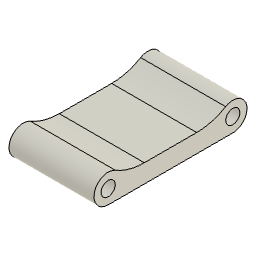
wing frame with feathers [both L + R] (Autodesk Fusion 360 archive; units mm, degrees)
design "pivots"
Autodesk Fusion 360 part; units mm, degrees
sketch "Sketch1" plane through (0, 0, 0) normal (1, 0, 0) x (0, 1, 0)
  line L0 (0, 0) -> (17, 0)
  circle A0 centre (20, 2.5) radius 1.25
  line L1 (-2, 0) -> (20, 0)
  line L2 (13.6213, 3.25) -> (4.3787, 3.25)
  arc A1 (-0.7243, 4.65) -> (-2, 0) centre (-2, 2.5) ccw
  arc A2 (20, 0) -> (18.7243, 4.65) centre (20, 2.5) ccw
  arc A3 (-0.7243, 4.65) -> (4.3787, 3.25) centre (4.3787, 13.25) ccw
  arc A4 (13.6213, 3.25) -> (18.7243, 4.65) centre (13.6213, 13.25) ccw
  circle A5 centre (-2, 2.5) radius 1.25
  dimension "d1" = 17
  dimension "d7" = 2.5
  dimension "d8" = 10
  dimension "d11" = 2.5
  constraint horizontal L0
  constraint coincident L0.start origin
  constraint concentric A0 A2
  constraint tangent L1 A2
  constraint parallel L0 L1
  constraint tangent L2 A3
  constraint tangent A1 A3
  constraint tangent L2 A4
  constraint tangent A2 A4
  constraint equal A3 A4
  constraint concentric A1 A5
  measures "d1" distance of L0.start L0.end
  measures "d7" diameter of A0
  measures "d8" radius of A3
  measures "d11" diameter of A5
extrude "Extrude1" add sketch "Sketch1" along normal blind 20 contours L0 L1 L2 A1 A2 A3 A4 | A0 | A5
extrude "Extrude2" cut sketch "Sketch1" along normal blind 50 contours A0
extrude "Extrude3" cut sketch "Sketch1" along normal blind 25.474 contours A5
extrude "Extrude4" cut 1 faces at (20, 7.4596, 1.0833) along direction (-1, 0, 0) blind 5
equation "d1 = 2 mm + 13 mm + 2 mm"

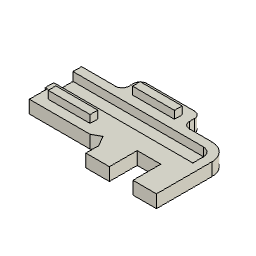
design "Right Shoulder Top"
Autodesk Fusion 360 part; units mm, degrees
sketch "Sketch1" plane through (0, 0, 0) normal (0, 0, 1) x (1, 0, 0)
  line L0 (0, 0) -> (20, 0)
  line L1 (20, 0) -> (20, 4.5)
  line L2 (20, 4.5) -> (0, 4.5)
  line L3 (0, 4.5) -> (0, 0)
  line L4 (20, 0) -> (21.5, 0)
  line L5 (21.5, 0) -> (21.5, 15)
  line L6 (21.5, 15) -> (20, 15)
  line L7 (20, 15) -> (20, 0)
  line L8 (31, 0) -> (32.5, 0)
  line L9 (32.5, 0) -> (32.5, 15)
  line L10 (32.5, 15) -> (31, 15)
  line L11 (31, 15) -> (31, 0)
  line L12 (20, 4.5) -> (16, 4.5)
  line L13 (16, 4.5) -> (16, 11.5)
  line L14 (16, 11.5) -> (20, 11.5)
  line L15 (20, 11.5) -> (20, 4.5)
  line L16 (21.5, 0) -> (31, 0)
  line L17 (31, 0) -> (31, 4.5)
  line L18 (31, 4.5) -> (21.5, 4.5)
  line L19 (21.5, 4.5) -> (21.5, 0)
  line L20 (21.5, 4.5) -> (31, 4.5)
  line L21 (31, 4.5) -> (31, 9.5)
  line L22 (31, 9.5) -> (21.5, 9.5)
  line L23 (21.5, 9.5) -> (21.5, 4.5)
  line L24 (81, 15) -> (81, 9.5)
  line L25 (50, 0) -> (70, 0)
  line L26 (71.5, 15) -> (70, 15)
  line L27 (50, 4.5) -> (50, 0)
  line L28 (66, 4.5) -> (50, 4.5)
  line L29 (82.5, 2) -> (82.5, 15)
  line L30 (71.5, 0) -> (80.5, 0)
  line L31 (82.5, 15) -> (81, 15)
  line L32 (70, 15) -> (70, 11.5)
  line L33 (70, 0) -> (71.5, 0)
  line L34 (71.5, 9.5) -> (71.5, 15)
  line L35 (66, 4.5) -> (70, 11.5)
  line L36 (71.5, 9.5) -> (71.5, 6.5)
  line L37 (71.5, 6.5) -> (81, 6.5)
  line L38 (81, 6.5) -> (81, 9.5)
  arc A0 (80.5, 0) -> (82.5, 2) centre (80.5, 2) ccw
  line L39 (70, -2) -> (71.5, -2)
  arc A1 (80.5, -2) -> (84.5, 2) centre (80.5, 2) ccw
  line L40 (84.5, 2) -> (84.5, 15)
  line L41 (79, 15) -> (79, 9.5)
  line L42 (79, 8.5) -> (79, 9.5)
  line L43 (73.5, 8.5) -> (79, 8.5)
  line L44 (73.5, 9.5) -> (73.5, 8.5)
  line L45 (73.5, 9.5) -> (73.5, 15)
  line L46 (68, 15) -> (68, 12.0311)
  line L47 (66.6143, 9.6061) -> (68, 12.0311)
  line L48 (50, 6.5) -> (50, -2)
  line L49 (68, 15) -> (73.5, 15)
  line L50 (79, 15) -> (84.5, 15)
  line L51 (52.5, 6.5) -> (62.7, 6.5)
  line L52 (62.7, 6.5) -> (62.7, 8.7)
  line L53 (62.7, 8.7) -> (52.5, 8.7)
  line L54 (52.5, 8.7) -> (52.5, 6.5)
  line L55 (64.7, 10.7) -> (50.5, 10.7)
  line L56 (50.5, 10.7) -> (50.5, 6.5)
  line L57 (62.7, 6.5) -> (52.5, 6.5)
  line L58 (50.5, 6.5) -> (50, 6.5)
  line L59 (64.7, 10.7) -> (66.6143, 9.6061)
  line L60 (61.5, -2) -> (71.7, -2)
  line L61 (71.7, -2) -> (71.7, -4.2)
  line L62 (71.7, -4.2) -> (61.5, -4.2)
  line L63 (61.5, -4.2) -> (61.5, -2)
  line L64 (73.7, -3.5) -> (73.7, -4.7)
  line L65 (72.2, -6.2) -> (61, -6.2)
  line L66 (59.5, -4.7) -> (59.5, -3.5)
  line L67 (71.5, -2) -> (71.7, -2)
  line L68 (75.2, -2) -> (80.5, -2)
  line L69 (50, -2) -> (58, -2)
  line L70 (61.5, -2) -> (70, -2)
  arc A2 (75.2, -2) -> (73.7, -3.5) centre (75.2, -3.5) ccw
  arc A3 (72.2, -6.2) -> (73.7, -4.7) centre (72.2, -4.7) ccw
  arc A4 (59.5, -4.7) -> (61, -6.2) centre (61, -4.7) ccw
  arc A5 (59.5, -3.5) -> (58, -2) centre (58, -3.5) ccw
  line L71 (70, 15) -> (71.5, 15)
  line L72 (71.5, 15) -> (71.5, 11.5)
  line L73 (71.5, 11.5) -> (70, 11.5)
  line L74 (70, 11.5) -> (70, 15)
  line L75 (71.7, -2) -> (71.7, -4.2)
  line L76 (61.5, -2) -> (71.7, -2)
  line L77 (70, -2) -> (71.5, -2)
  line L78 (71.7, -4.2) -> (61.5, -4.2)
  line L79 (68, 15) -> (73.5, 15)
  line L80 (70, 15) -> (71.5, 15)
  line L81 (71.5, 11.5) -> (70, 11.5)
  line L82 (72.2, -6.2) -> (61, -6.2)
  line L83 (71.5, 15) -> (70, 15)
  line L84 (70, 0) -> (71.5, 0)
  line L85 (71.5, 9.5) -> (71.5, 15)
  line L86 (73.5, 8.5) -> (79, 8.5)
  line L87 (70, 15) -> (70, 11.5)
  line L88 (75.2, -2) -> (80.5, -2)
  line L89 (79, 8.5) -> (79, 9.5)
  line L90 (82.5, 15) -> (81, 15)
  line L91 (81, 15) -> (81, 9.5)
  line L92 (73.5, 9.5) -> (73.5, 8.5)
  line L93 (71.5, 6.5) -> (81, 6.5)
  arc A6 (75.2, -2) -> (73.7, -3.5) centre (75.2, -3.5) ccw
  arc A7 (80.5, -2) -> (84.5, 2) centre (80.5, 2) ccw
  line L94 (61.5, -2) -> (70, -2)
  line L95 (71.5, 15) -> (71.5, 11.5)
  line L96 (52.5, 8.7) -> (52.5, 6.5)
  line L97 (52.5, 6.5) -> (62.7, 6.5)
  line L98 (79, 15) -> (79, 9.5)
  line L99 (68, 15) -> (68, 12.0311)
  line L100 (82.5, 2) -> (82.5, 15)
  line L101 (66, 4.5) -> (50, 4.5)
  line L102 (79, 15) -> (84.5, 15)
  line L103 (50, 4.5) -> (50, 0)
  line L104 (64.7, 10.7) -> (66.6143, 9.6061)
  line L105 (73.5, 9.5) -> (73.5, 15)
  line L106 (50.5, 10.7) -> (50.5, 6.5)
  line L107 (50, 0) -> (70, 0)
  line L108 (84.5, 2) -> (84.5, 15)
  line L109 (59.5, -4.7) -> (59.5, -3.5)
  line L110 (71.5, -2) -> (71.7, -2)
  line L111 (61.5, -4.2) -> (61.5, -2)
  line L112 (73.7, -3.5) -> (73.7, -4.7)
  line L113 (50, 6.5) -> (50, -2)
  line L114 (71.5, 0) -> (80.5, 0)
  arc A8 (59.5, -4.7) -> (61, -6.2) centre (61, -4.7) ccw
  line L115 (81, 6.5) -> (81, 9.5)
  arc A9 (59.5, -3.5) -> (58, -2) centre (58, -3.5) ccw
  line L116 (62.7, 8.7) -> (52.5, 8.7)
  arc A10 (72.2, -6.2) -> (73.7, -4.7) centre (72.2, -4.7) ccw
  line L117 (70, 11.5) -> (70, 15)
  arc A11 (80.5, 0) -> (82.5, 2) centre (80.5, 2) ccw
  line L118 (50.5, 6.5) -> (50, 6.5)
  line L119 (66.6143, 9.6061) -> (68, 12.0311)
  line L120 (71.5, 9.5) -> (71.5, 6.5)
  line L121 (62.7, 6.5) -> (52.5, 6.5)
  line L122 (64.7, 10.7) -> (50.5, 10.7)
  line L123 (50, -2) -> (58, -2)
  line L124 (62.7, 6.5) -> (62.7, 8.7)
  line L125 (66, 4.5) -> (70, 11.5)
  line L126 (50, 42) -> (58, 42)
  line L127 (66.6143, 30.3939) -> (68, 27.9689)
  line L128 (50.5, 33.5) -> (50, 33.5)
  line L129 (50, 33.5) -> (50, 42)
  line L130 (64.7, 29.3) -> (66.6143, 30.3939)
  line L131 (64.7, 29.3) -> (50.5, 29.3)
  line L132 (68, 25) -> (68, 27.9689)
  line L133 (50, 40) -> (70, 40)
  line L134 (50, 35.5) -> (50, 40)
  line L135 (50.5, 33.5) -> (50, 33.5)
  line L136 (50, 42) -> (58, 42)
  arc A12 (61, 46.2) -> (59.5, 44.7) centre (61, 44.7) ccw
  line L137 (64.7, 29.3) -> (50.5, 29.3)
  arc A13 (58, 42) -> (59.5, 43.5) centre (58, 43.5) ccw
  line L138 (50.5, 29.3) -> (50.5, 33.5)
  line L139 (59.5, 44.7) -> (59.5, 43.5)
  line L140 (73.5, 30.5) -> (73.5, 25)
  line L141 (70, 40) -> (71.5, 40)
  line L142 (79, 31.5) -> (79, 30.5)
  line L143 (50, 33.5) -> (50, 42)
  line L144 (71.5, 40) -> (80.5, 40)
  line L145 (66.6143, 30.3939) -> (68, 27.9689)
  line L146 (66, 35.5) -> (50, 35.5)
  line L147 (64.7, 29.3) -> (66.6143, 30.3939)
  arc A14 (82.5, 38) -> (80.5, 40) centre (80.5, 38) ccw
  line L148 (50, 35.5) -> (50, 40)
  line L149 (50, 40) -> (70, 40)
  line L150 (84.5, 38) -> (84.5, 25)
  line L151 (79, 25) -> (84.5, 25)
  line L152 (79, 25) -> (79, 30.5)
  line L153 (68, 25) -> (73.5, 25)
  line L154 (73.5, 31.5) -> (79, 31.5)
  line L155 (79, 25) -> (79, 30.5)
  line L156 (70, 25) -> (71.5, 25)
  line L157 (68, 25) -> (73.5, 25)
  line L158 (71.5, 25) -> (70, 25)
  line L159 (75.2, 42) -> (80.5, 42)
  line L160 (70, 25) -> (71.5, 25)
  arc A15 (73.7, 44.7) -> (72.2, 46.2) centre (72.2, 44.7) ccw
  arc A16 (84.5, 38) -> (80.5, 42) centre (80.5, 38) ccw
  line L161 (73.7, 43.5) -> (73.7, 44.7)
  line L162 (73.5, 30.5) -> (73.5, 31.5)
  line L163 (73.5, 30.5) -> (73.5, 31.5)
  line L164 (79, 25) -> (84.5, 25)
  line L165 (82.5, 25) -> (81, 25)
  arc A17 (73.7, 43.5) -> (75.2, 42) centre (75.2, 43.5) ccw
  line L166 (73.7, 43.5) -> (73.7, 44.7)
  line L167 (71.5, 40) -> (80.5, 40)
  line L168 (79, 31.5) -> (79, 30.5)
  line L169 (71.5, 25) -> (70, 25)
  line L170 (82.5, 25) -> (81, 25)
  line L171 (75.2, 42) -> (80.5, 42)
  line L172 (70, 40) -> (71.5, 40)
  line L173 (72.2, 46.2) -> (61, 46.2)
  line L174 (73.5, 31.5) -> (79, 31.5)
  line L175 (73.5, 30.5) -> (73.5, 25)
  line L176 (72.2, 46.2) -> (61, 46.2)
  arc A18 (73.7, 43.5) -> (75.2, 42) centre (75.2, 43.5) ccw
  arc A19 (58, 42) -> (59.5, 43.5) centre (58, 43.5) ccw
  arc A20 (82.5, 38) -> (80.5, 40) centre (80.5, 38) ccw
  arc A21 (84.5, 38) -> (80.5, 42) centre (80.5, 38) ccw
  line L177 (68, 25) -> (68, 27.9689)
  arc A22 (73.7, 44.7) -> (72.2, 46.2) centre (72.2, 44.7) ccw
  line L178 (59.5, 44.7) -> (59.5, 43.5)
  line L179 (50.5, 29.3) -> (50.5, 33.5)
  arc A23 (61, 46.2) -> (59.5, 44.7) centre (61, 44.7) ccw
  line L180 (66, 35.5) -> (50, 35.5)
  line L181 (84.5, 38) -> (84.5, 25)
  line L182 (52.7, 31.5) -> (52.7, 33.3)
  line L183 (62.5, 33.3) -> (52.7, 33.3)
  line L184 (62.5, 33.3) -> (62.5, 31.5)
  line L185 (62.5, 31.5) -> (52.7, 31.5)
  line L186 (71.5, 42.2) -> (71.5, 44)
  line L187 (71.5, 44) -> (61.7, 44)
  line L188 (61.7, 44) -> (61.7, 42.2)
  line L189 (61.7, 42.2) -> (71.5, 42.2)
  line L190 (66, 35.5) -> (82.5, 35.5)
  line L191 (82.5, 38) -> (82.5, 35.5)
  point P0 (50, 0)
  point P1 (50, 0)
  point P2 (50, 40)
  point P3 (50, 40)
  dimension "d1" = 20
  dimension "d2" = 4.5
  dimension "d3" = 1.5
  dimension "d4" = 15
  dimension "d5" = 1.5
  dimension "d6" = 15
  dimension "d7" = 9.5
  dimension "d8" = 4
  dimension "d9" = 7
  dimension "d10" = 4.5
  dimension "d27" = 2
  dimension "d29" = 10.2
  dimension "d30" = 2.2
  dimension "d32" = 10.2
  dimension "d33" = 2.2
  dimension "d35" = 1.5
  dimension "d36" = 3.5
  dimension "d43" = 2
  dimension "d44" = 10.2
  dimension "d45" = 2.2
  dimension "d46" = 10.2
  dimension "d47" = 2.2
  dimension "d48" = 1.5
  dimension "d49" = 3.5
  constraint horizontal L0
  constraint vertical L1
  constraint horizontal L2
  constraint vertical L3
  constraint coincident L0.start L3.end
  constraint horizontal L4
  constraint vertical L5
  constraint horizontal L6
  constraint vertical L7
  constraint horizontal L8
  constraint vertical L9
  constraint horizontal L10
  constraint vertical L11
  constraint horizontal L12
  constraint vertical L13
  constraint horizontal L14
  constraint vertical L15
  constraint horizontal L16
  constraint vertical L17
  constraint horizontal L18
  constraint vertical L19
  constraint horizontal L20
  constraint vertical L21
  constraint horizontal L22
  constraint vertical L23
  constraint coincident L11 L21.end
  constraint horizontal L25
  constraint horizontal L28
  constraint vertical L27
  constraint coincident P1 P0
  constraint horizontal L33
  constraint vertical L34
  constraint horizontal L26
  constraint vertical L32
  constraint vertical L29
  constraint horizontal L31
  constraint vertical L24
  constraint horizontal L30
  constraint perpendicular L36 L37
  constraint tangent L29 A0
  constraint perpendicular L46 L49
  constraint concentric A0 A1
  constraint tangent A1 L40
  constraint tangent A1 L67
  constraint coincident L41.start L49
  constraint collinear L49 L50
  constraint horizontal L51
  constraint vertical L52
  constraint horizontal L53
  constraint vertical L54
  constraint collinear L57 L58
  constraint perpendicular L47 L59
  constraint horizontal L60
  constraint vertical L61
  constraint horizontal L62
  constraint vertical L63
  constraint coincident L60.start L69
  constraint collinear L67 L68
  constraint collinear L69 L70
  constraint tangent L64 A2
  constraint tangent L68 A2
  constraint tangent L64 A3
  constraint tangent L65 A3
  constraint equal A2 A3
  constraint tangent L65 A4
  constraint tangent L66 A4
  constraint equal A2 A4
  constraint tangent L66 A5
  constraint tangent L69 A5
  constraint equal A2 A5
  constraint horizontal L71
  constraint vertical L72
  constraint horizontal L73
  constraint vertical L74
  constraint coincident L34 L72.end
  constraint horizontal L107
  constraint horizontal L101
  constraint vertical L103
  constraint horizontal L84
  constraint vertical L85
  constraint horizontal L83
  constraint vertical L87
  constraint vertical L100
  constraint horizontal L90
  constraint vertical L91
  constraint horizontal L114
  constraint perpendicular L93 L120
  constraint tangent L100 A11
  constraint perpendicular L79 L99
  constraint concentric A7 A11
  constraint tangent A7 L108
  constraint tangent A7 L110
  constraint coincident L41.start L79
  constraint collinear L79 L102
  constraint horizontal L97
  constraint vertical L124
  constraint horizontal L116
  constraint vertical L96
  constraint collinear L118 L121
  constraint perpendicular L104 L119
  constraint horizontal L76
  constraint vertical L75
  constraint horizontal L78
  constraint vertical L111
  constraint coincident L60.start L123
  constraint collinear L88 L110
  constraint collinear L94 L123
  constraint tangent A6 L112
  constraint tangent L88 A6
  constraint tangent L112 A10
  constraint tangent L82 A10
  constraint equal A6 A10
  constraint tangent L82 A8
  constraint tangent L109 A8
  constraint equal A6 A8
  constraint tangent L109 A9
  constraint tangent A9 L123
  constraint equal A6 A9
  constraint horizontal L80
  constraint vertical L95
  constraint horizontal L81
  constraint vertical L117
  constraint coincident L72.end L85
  constraint parallel L146 L190
  measures "d1" distance of L0.start L0.end
  measures "d2" distance of L0.start L2.end
  measures "d3" distance of L0.end L4.end
  measures "d4" distance of L0.end L6.end
  measures "d5" distance of L8.start L8.end
  measures "d6" distance of L8.start L10.end
  measures "d7" distance of L5 L11
  measures "d8" distance of L1.end L12.end
  measures "d9" distance of L1.end L14.end
  measures "d10" distance of L4.end L18.end
  measures "d27" radius of A0
  measures "d29" distance of L51.start L51.end
  measures "d30" distance of L51.start L53.end
  measures "d32" distance of L60.start L60.end
  measures "d33" distance of L60.start L62.end
  measures "d35" radius of A2
  measures "d36" distance of L26.end L32.end
  measures "d43" radius of A11
  measures "d44" distance of L51.start L51.end
  measures "d45" distance of L51.start L53.end
  measures "d46" distance of L60.start L60.end
  measures "d47" distance of L62.end L60.start
  measures "d48" radius of A6
  measures "d49" distance of L26.end L32.end
extrude "Extrude6" add sketch "Sketch1" against normal blind 3 contours L126 L127 L128 L129 L130 L131 L132 L133 L135 L136 A12 L137 A13 L138 L139 L140 L141 L142 L143 L144 L145 L146 L147 A14 L149 L150 L151 L152 L153 L154 L155 L156 L157 L158 L159 L160 A15 A16 L161 L162 L163 L164 L165 A17 L166 L167 L168 L169 L170 L171 L172 L173 L174 L175 L176 A18 A19 A20 A21 L177 A22 L178 L179 A23 L180 L181 L190 L191 | L129 L133 L134 L141 L143 L144 L146 A14 L148 L149 L167 L172 A20 L180 L190 L191 | L182 L183 L184 L185 | L186 L187 L188 L189
extrude "Extrude7" add sketch "Sketch1" along normal blind 1.8 contours L182 L183 L184 L185 | L186 L187 L188 L189
extrude "Extrude8" cut sketch "Sketch1" against normal blind 2 contours L129 L133 L134 L141 L143 L144 L146 A14 L148 L149 L167 L172 A20 L180 L190 L191
ref_plane "WorkPlane1" through (95.211, 0, 0) normal (1, 0, 0) x (0, 1, 0)
extrude "Extrude10" cut 1 faces at (50.0003, 37.0002, -0.6666) along direction (-1, 0, 0) blind 10
